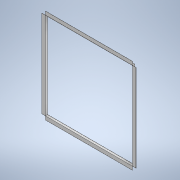
# Autodesk Inventor part: Fastening Frame
Saved by Autodesk Inventor 2022 (Build 260153000, 153)
## iProperties
Created: 2022-03-06
Part Number: Fastening Frame
Material: Generic
Document SubType Name: Modeling
Designer: calvi
Density: 1 g/cm^3
Appearance: Default
Author: calvi
Autodesk Inventor part; units mm, degrees
ref_plane "YZ Plane" through (0, 0, 0) normal (1, 0, 0) x (0, 1, 0)
ref_plane "XZ Plane" through (0, 0, 0) normal (0, 1, 0) x (-1, 0, 0)
ref_plane "XY Plane" through (0, 0, 0) normal (0, 0, 1) x (1, 0, 0)
sketch "Sketch1" plane through (0, 0, 0) normal (0, 0, 1) x (1, 0, 0)
  line L0 (604.25, 605) -> (604.25, -605)
  line L1 (604.25, -605) -> (-604.25, -605)
  line L2 (-604.25, -605) -> (-604.25, 605)
  line L3 (-604.25, 605) -> (604.25, 605)
  line L4 (605.75, -606.5) -> (-605.75, -606.5)
  line L5 (605.75, 606.5) -> (605.75, -606.5)
  line L6 (-605.75, 606.5) -> (605.75, 606.5)
  line L7 (-605.75, -606.5) -> (-605.75, 606.5)
  line L8 (-605.75, 606.5) -> (-655.75, 606.5)
  line L9 (-655.75, 606.5) -> (-655.75, -606.5)
  line L10 (-655.75, -606.5) -> (-605.75, -606.5)
  line L11 (-605.75, -606.5) -> (-605.75, 606.5)
  line L12 (-605.75, -606.5) -> (605.75, -606.5)
  line L13 (605.75, -606.5) -> (605.75, -656.5)
  line L14 (605.75, -656.5) -> (-605.75, -656.5)
  line L15 (-605.75, -656.5) -> (-605.75, -606.5)
  line L16 (605.75, -606.5) -> (655.75, -606.5)
  line L17 (655.75, -606.5) -> (655.75, 606.5)
  line L18 (655.75, 606.5) -> (605.75, 606.5)
  line L19 (605.75, 606.5) -> (605.75, -606.5)
  line L20 (605.75, 606.5) -> (-605.75, 606.5)
  line L21 (-605.75, 606.5) -> (-605.75, 656.5)
  line L22 (-605.75, 656.5) -> (605.75, 656.5)
  line L23 (605.75, 656.5) -> (605.75, 606.5)
  point P0 (0, 0)
  point P1 (0, 0)
  point P2 (-605.75, -606.5)
  point P3 (-605.75, -606.5)
  point P4 (-605.75, -606.5)
  point P5 (-605.75, -606.5)
  dimension "d0" = 50
  dimension "d1" = 50
  dimension "d2" = 50
  dimension "d3" = 50
  constraints: 48 end point, 8 parallel, 4 horizontal, 4 perpendicular, 2 point on line
  measures "d0" distance of L10.end L9.end
  measures "d1" distance of L12.end L13.end
  measures "d2" distance of L18.end L17.end
  measures "d3" distance of L20.end L21.end
extrude "Extrusion1" add sketch "Sketch1" along normal blind 1.5 contours L13 L14 L15 L4 | L5 L18 L17 L16 | L10 L9 L8 L7 | L6 L21 L22 L23
sketch "Sketch2" plane through (0, 0, 0) normal (0, 0, -1) x (-1, 0, 0)
  line L0 (-605.75, 606.5) -> (-605.75, -606.5) projected
  line L1 (-605.75, -606.5) -> (605.75, -606.5) projected
  line L2 (-605.75, 606.5) -> (605.75, 606.5)
  line L3 (605.75, 606.5) -> (605.75, -606.5)
  line L4 (605.75, -606.5) -> (-605.75, -606.5)
  line L5 (-605.75, -606.5) -> (-605.75, 606.5)
  line L6 (607.25, 608) -> (-607.25, 608)
  line L7 (-607.25, 608) -> (-607.25, -608)
  line L8 (-607.25, -608) -> (607.25, -608)
  line L9 (607.25, -608) -> (607.25, 608)
  point P0 (0, 0)
  dimension "d6" = 1.5
  constraints: 16 end point, 4 parallel, 2 perpendicular, 1 horizontal, 3 other
  measures "d6" distance between parallel lines of L2 L6
extrude "Extrusion2" add sketch "Sketch2" along normal blind 30
body "Solid1"
